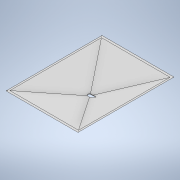
# Autodesk Inventor part: newconeholder
Saved by Autodesk Inventor 2021 (Build 250183000, 183)
## iProperties
Created: 2021-11-17
Part Number: newconeholder
Material: Generic
Document SubType Name: Modeling
Designer: mattc
Density: 1 g/cm^3
Appearance: Default
Author: mattc
Autodesk Inventor part; units mm, degrees
ref_plane "YZ Plane" through (0, 0, 0) normal (1, 0, 0) x (0, 1, 0)
ref_plane "XZ Plane" through (0, 0, 0) normal (0, 1, 0) x (-1, 0, 0)
ref_plane "XY Plane" through (0, 0, 0) normal (0, 0, 1) x (1, 0, 0)
sketch "cone top" plane through (0, 0, 0) normal (0, 1, 0) x (-1, 0, 0)
  line L0 (-7.5, 10) -> (7.5, 10)
  line L1 (7.5, 10) -> (7.5, -10)
  line L2 (7.5, -10) -> (-7.5, -10)
  line L3 (-7.5, -10) -> (-7.5, 10)
  line L4 (-7.5, 10) -> (7.5, -10) construction
  line L5 (7.5, 10) -> (-7.5, -10) construction
  point P0 (0, 0)
  dimension "d0" = 15
  dimension "d1" = 20
  constraints: 12 end point, 2 midpoint, 2 parallel, 1 horizontal, 1 perpendicular
  measures "d0" distance of L1.end L2.end
  measures "d1" distance of L0.end L1.end
ref_plane "Work Plane2" through (0, -2.25, 0) normal (0, 1, 0) x (-1, 0, 0)
sketch "fly slot" plane through (0, -2.25, 0) normal (0, 1, 0) x (-1, 0, 0)
  spline S0 degree 4 poles (0.3964, -0.0002) (0.3991, -0.0499) (0.4019, -0.1475) (0.3162, -0.3523) (0.1925, -0.3295) (-0.2287, -0.3672) (-0.6422, -0.361) (-1.2582, -0.0137) (-1.2268, -0.0002) knots 0 0 0 0 0 0.11031 0.216226 0.372169 0.55077 1 1 1 1 1
  line L0 (0.3964, -0.0002) -> (-1.2268, -0.0002)
  spline S1 degree 4 poles (0.3964, -0.0002) (0.3937, 0.0489) (0.3859, 0.145) (0.3272, 0.3535) (0.185, 0.3281) (-0.2182, 0.3684) (-0.6512, 0.3594) (-1.2552, 0.0138) (-1.2268, -0.0002) knots 0 0 0 0 0 0.11031 0.216226 0.372169 0.55077 1 1 1 1 1
  point P0 (0.3234, -0.2856)
  point P1 (0.2125, -0.337)
  point P2 (-0.4465, -0.3294)
  point P3 (-1.1043, -0.0852)
  point P4 (-0.0232, -0.3469)
  point P5 (0.3234, 0.2853)
  point P6 (0.2125, 0.3367)
  point P7 (-0.4465, 0.3291)
  point P8 (-1.1043, 0.0849)
  point P9 (-0.0232, 0.3466)
  constraints: 5 symmetric about line, 2 end point, 14 other
sketch "Sketch6" plane through (0, -2.25, 0) normal (0, 1, 0) x (-1, 0, 0)
  line L0 (-0.0165, -0.0313) -> (0.0165, -0.0313)
  line L1 (0.0165, -0.0313) -> (0.0165, 0.0313)
  line L2 (0.0165, 0.0313) -> (-0.0165, 0.0313)
  line L3 (-0.0165, 0.0313) -> (-0.0165, -0.0313)
  line L4 (-0.0165, -0.0313) -> (0.0165, 0.0313) construction
  line L5 (0.0165, -0.0313) -> (-0.0165, 0.0313) construction
  point P0 (0, 0)
  constraints: 12 end point, 2 midpoint, 2 parallel, 1 horizontal, 1 perpendicular
loft "Loft3" add profiles "cone top", "Sketch6"
shell "Shell1" thickness 0.1 removed faces 1 at (2.5, 0, 3.3333)
extrude "Extrusion4" cut sketch "fly slot" along normal blind 10
body "Solid4"
